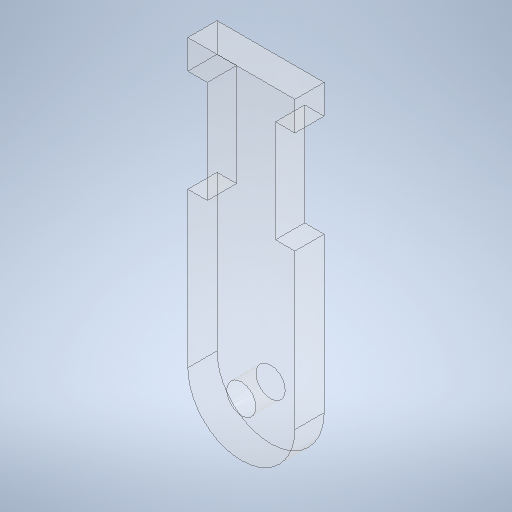
# Autodesk Inventor part: 4P.01.01.16-BC-v1-Final Flap L2 80deg
Saved by Autodesk Inventor 2025.2 (Build 292293000, 293)
## iProperties
Category: <PART CATAGORY>
Created: 2025-01-30
Part Number: 4P.01.01.16-BC-v1-Final Flap L2 80deg
Material: Acrylic, Clear
Document SubType Name: Modeling
Designer: Carriett 4
Density: 1.19 g/cm^3
Appearance: Transparent - Clear
Title: <TITLE>
Author: Carriett 4
Revision Number: 1
Autodesk Inventor part; units mm, degrees
ref_plane "YZ Plane" through (0, 0, 0) normal (1, 0, 0) x (0, 1, 0)
ref_plane "XZ Plane" through (0, 0, 0) normal (0, 1, 0) x (-1, 0, 0)
ref_plane "XY Plane" through (0, 0, 0) normal (0, 0, 1) x (1, 0, 0)
sketch "Sketch6" plane through (0, 0, 0) normal (0, 0, 1) x (1, 0, 0)
  line L0 (11, 34.8851) -> (0, 34.8851)
  line L1 (2, 31.8851) -> (2, 21.3851)
  line L2 (9, 31.8851) -> (9, 21.3851)
  line L3 (2, 21.3851) -> (0, 21.3851)
  line L4 (9, 21.3851) -> (11, 21.3851)
  arc A0 (0, 5.5) -> (11, 5.5) centre (5.5, 5.5) ccw
  circle A1 centre (5.5, 5.5) radius 1.5
  line L5 (0, 31.8851) -> (2, 31.8851)
  line L6 (9, 31.8851) -> (11, 31.8851)
  line L7 (0, 34.8851) -> (0, 31.8851)
  line L8 (0, 21.3851) -> (0, 5.5)
  line L9 (11, 5.5) -> (11, 21.3851)
  line L10 (11, 31.8851) -> (11, 34.8851)
  point P0 (0, 0)
  point P1 (10, 21.3851)
  dimension "d92" = 10.5
  dimension "d93" = 10.5
  dimension "d94" = 2
  dimension "d95" = 2
  dimension "d96" = 3
  dimension "d97" = 11
  dimension "d98" = 15.8851
  constraints: 22 end point, 6 perpendicular, 4 parallel, 4 tangent, 2 centre point, 2 point on circle, 2 vertical, 1 coincident, 1 midpoint, 1 point on line
  measures "d92" distance between parallel lines of L4 L6
  measures "d93" distance between parallel lines of L5 L3
  measures "d94" distance between parallel lines of L1 L7
  measures "d95" distance between parallel lines of L10 L2
  measures "d96" distance of L0.end L5.start
  measures "d97" distance between parallel lines of L10 L7
  measures "d98" vertical distance of A0.centre point (10, 21.385)
extrude "Extrusion3" add sketch "Sketch6" along normal blind 3
body "Solid2"
